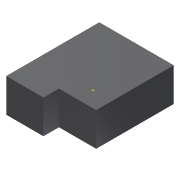
# Autodesk Inventor part: data
Saved by Autodesk Inventor 2015 (Build 190159000, 159)
## iProperties
Created: 2021-06-10
Part Number: data
Material: ABS Plastic
Document SubType Name: Modeling
Designer: Mia
Density: 1.06 g/cm^3
Appearance: Textured - Gray
Author: Mia
Autodesk Inventor part; units mm, degrees
ref_plane "YZ Plane" through (0, 0, 0) normal (1, 0, 0) x (0, 1, 0)
ref_plane "XZ Plane" through (0, 0, 0) normal (0, 1, 0) x (-1, 0, 0)
ref_plane "XY Plane" through (0, 0, 0) normal (0, 0, 1) x (1, 0, 0)
ref_plane "Work Plane1" through (0, 0, 0) normal (0, 0, 1) x (1, 0, 0)
sketch "Sketch2" plane through (0, 0, 0) normal (0, 0, 1) x (1, 0, 0)
  line L0 (-900, -1000) -> (900, -1000) projected
  line L1 (900, -1000) -> (900, 1000) projected
  line L2 (900, 1000) -> (-900, 1000) projected
  line L3 (-900, 1000) -> (-900, -1000) projected
  line L4 (900, -1000) -> (-900, -1000) projected
  line L5 (-900, -1000) -> (-900, -500)
  line L6 (-900, -1000) -> (-900, 1000) projected
  line L7 (-300, -500) -> (-300, -250)
  line L8 (-300, -250) -> (300, -250)
  line L9 (300, -250) -> (300, 1000)
  line L10 (-900, 1000) -> (-900, -500)
  line L11 (-300, -500) -> (-900, -500)
  point P0 (0, 0)
  point P1 (-300, -1000)
  point P2 (300, -1000)
  dimension "d4" = 600
  dimension "d5" = 600
  dimension "d6" = 600
  dimension "d7" = 500
  dimension "d8" = 1200
  dimension "d9" = 750
  dimension "d10" = 1500
  constraints: 12 end point, 4 point on line, 2 perpendicular, 1 collinear, 1 vertical
  measures "d4" distance from line of L3 point (-300, -1000)
  measures "d5" distance of point (-300, -1000) point (300, -1000)
  measures "d6" distance from line of L3 L7.start
  measures "d7" distance from line of L0 L7.start
  measures "d8" distance from line of L3 L8.end
  measures "d9" distance from line of L0 L8.end
  measures "d10" distance from line of L5.end L2
extrude "Extrusion2" [suppressed]
ref_plane "Work Plane2" through (0, 0, 0) normal (0, 0, 1) x (1, 0, 0)
sketch "Sketch4" plane through (0, 0, 0) normal (0, 0, 1) x (1, 0, 0)
  line L0 (-300, -500) -> (-900, -500) projected
  line L1 (-900, -500) -> (-900, -1000) projected
  line L2 (-900, -1000) -> (900, -1000) projected
  line L3 (900, -1000) -> (900, 1000) projected
  line L4 (900, 1000) -> (300, 1000) projected
  line L5 (300, 1000) -> (300, -250) projected
  line L6 (300, -250) -> (-300, -250) projected
  line L7 (-300, -250) -> (-300, -500) projected
  line L8 (300, 1000) -> (300, -250)
  line L9 (300, -250) -> (-300, -250)
  line L10 (-300, -500) -> (-900, -500)
  line L11 (-300, -500) -> (-300, -250) projected
  line L12 (-900, 1000) -> (300, 1000)
  line L13 (-900, 1000) -> (-900, -500)
  point P0 (0, 0)
  constraints: 10 end point, 2 perpendicular, 2 vertical, 1 collinear
extrude "Extrusion4" add sketch "Sketch4" against normal blind 540 contours L0 L13 L12 L5 L6 L7
body "Solid1"
